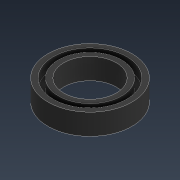
# Autodesk Inventor part: Uszczelka front
Saved by Autodesk Inventor 2022 (Build 260153000, 153)
## iProperties
Created: 2023-04-12
Part Number: Uszczelka front
Material: Rubber
Document SubType Name: Modeling
Designer: wikto
Density: 0.93 g/cm^3
Appearance: Rubber - Black
Author: wikto
Autodesk Inventor part; units mm, degrees
ref_plane "YZ Plane" through (0, 0, 0) normal (1, 0, 0) x (0, 1, 0)
ref_plane "XZ Plane" through (0, 0, 0) normal (0, 1, 0) x (-1, 0, 0)
ref_plane "XY Plane" through (0, 0, 0) normal (0, 0, 1) x (1, 0, 0)
sketch "Sketch1" plane through (0, 0, 0) normal (0, 1, 0) x (-1, 0, 0)
  circle A0 centre (0, 0) radius 10
  circle A1 centre (0, 0) radius 12
  circle A2 centre (0, 0) radius 14
  circle A3 centre (0, 0) radius 16
  dimension "d0" = 20
  dimension "d1" = 24
  dimension "d2" = 32
  dimension "d3" = 28
  constraints: 4 centre point, 4 coincident
  measures "d0" diameter of A0
  measures "d1" diameter of A1
  measures "d2" diameter of A3
  measures "d3" diameter of A2
extrude "Extrusion1" add sketch "Sketch1" along normal blind 8
extrude "Extrusion2" add sketch "Sketch1" along normal blind 4 contours A2
body "Solid1"
